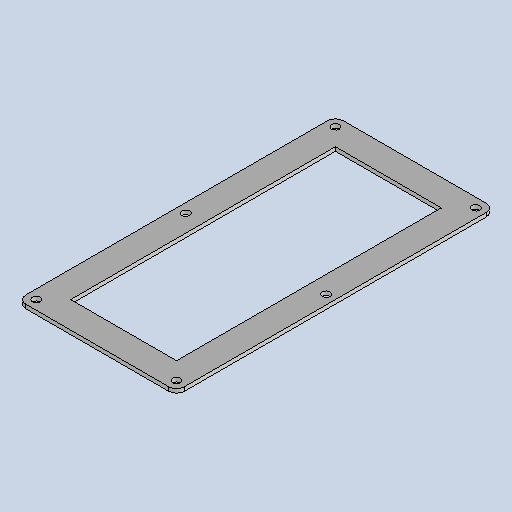
# Autodesk Inventor part: TKS 3521 BOTTOM FDS Diam way flange 1
Saved by Autodesk Inventor 2025 (Build 290162010, 162A)
## iProperties
Created: 2025-06-24
Part Number: TKS 3521 BOTTOM FDS Diam way flange 1
Material: Stainless Steel
Document SubType Name: Sheet Metal
Designer: admin
Mass: 103.446 g
Surface Area: 101.897 cm^2
Volume: 12.9307 cm^3
Density: 8 g/cm^3
Flat Pattern Width: 12 cm
Flat Pattern Length: 24 cm
Flat Pattern Area: 288 cm^2
Sheet Metal Rule: AISI304 2mm Die16
Sheet Metal Width: 120,000 mm
Sheet Metal Length: 240,000 mm
Sheet Metal Area: 28800,000 mm^2
Appearance: Default
Author: user
Autodesk Inventor part; units mm, degrees
ref_plane "YZ Plane" through (0, 0, 0) normal (1, 0, 0) x (0, 1, 0)
ref_plane "XZ Plane" through (0, 0, 0) normal (0, 1, 0) x (-1, 0, 0)
ref_plane "XY Plane" through (0, 0, 0) normal (0, 0, 1) x (1, 0, 0)
sketch "Sketch1" plane through (0, 0, 0) normal (0, 0, 1) x (1, 0, 0)
  line L0 (-60, -120) -> (60, -120)
  line L1 (60, -120) -> (60, 120)
  line L2 (60, 120) -> (-60, 120)
  line L3 (-60, 120) -> (-60, -120)
  line L4 (-60, -120) -> (60, 120) construction
  line L5 (60, -120) -> (-60, 120) construction
  line L6 (40, -100) -> (-40, -100)
  line L7 (-40, -100) -> (-40, 100)
  line L8 (-40, 100) -> (40, 100)
  line L9 (40, 100) -> (40, -100)
  line L10 (40, -100) -> (-40, 100) construction
  line L11 (-40, -100) -> (40, 100) construction
  point P0 (0, 0)
  dimension "d172" = 80
  dimension "d180" = 20
  dimension "d181" = 20
  dimension "d182" = 200
  measures "d172" distance of L7.end L8.end
  measures "d180" distance between parallel lines of L3 L7
  measures "d181" distance between parallel lines of L8 L2
  measures "d182" distance of L6.end L7.end
extrude "Plate5" add sketch "Sketch1" along normal blind 3
sketch "Sketch9" plane through (0, 0, 3) normal (0, 0, 1) x (1, 0, 0)
  circle A0 centre (53, -113) radius 3
  line L0 (53, 113) -> (-53, 113) construction
  line L1 (-53, 113) -> (-53, -113) construction
  line L2 (-53, -113) -> (53, -113) construction
  line L3 (53, -113) -> (53, 113) construction
  line L4 (53, 113) -> (-53, -113) construction
  line L5 (-53, 113) -> (53, -113) construction
  circle A1 centre (-53, -113) radius 3
  circle A2 centre (53, 113) radius 3
  circle A3 centre (-53, 113) radius 3
  line L6 (-40, -100) -> (-40, 100) projected
  line L7 (-40, 100) -> (40, 100) projected
  line L8 (40, 100) -> (40, -100) projected
  line L9 (40, -100) -> (-40, -100) projected
  line L10 (60, -120) -> (-60, -120) projected
  line L11 (60, 120) -> (60, -120) projected
  line L12 (-60, 120) -> (60, 120) projected
  line L13 (-60, -120) -> (-60, 120) projected
  circle A4 centre (-53, 0) radius 3
  circle A5 centre (53, 0) radius 3
  point P0 (0, 0)
  dimension "d174" = 6
  dimension "d183" = 7
  dimension "d184" = 7
  constraints: 12 end point, 7 coincident, 6 centre point, 5 equal radius, 4 midpoint, 2 parallel, 1 horizontal, 1 perpendicular
  measures "d174" diameter of A0
  measures "d183" distance from line of L0.start L12
  measures "d184" distance from line of L0.start L11
extrude "Cut2" cut sketch "Sketch9" against normal blind 3 contours A0 | A1 | A2 | A3 | A4 | A5
fillet "Corner Round1" radius 6 4 edges at (60, 120, 1.5) (-60, 120, 1.5) (-60, -120, 1.5) (60, -120, 1.5)
body "Solid3"
